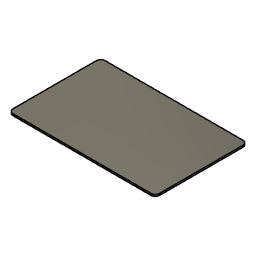
Part (Autodesk Fusion 360 archive; units mm, degrees)
design "Stainless_Steelx1mm_FacePlate"
Autodesk Fusion 360 part; units mm, degrees
sketch "Sketch1" plane through (0, 0, 0) normal (0, 1, 0) x (1, 0, 0)
  line L0 (40.5, -27) -> (-40.5, -27)
  line L1 (-43, -24.5) -> (-43, 24.5)
  line L2 (-40.5, 27) -> (40.5, 27)
  line L3 (43, 24.5) -> (43, -24.5)
  line L4 (43, -27) -> (-43, 27) construction
  line L5 (-43, -27) -> (43, 27) construction
  arc A0 (-40.5, 27) -> (-43, 24.5) centre (-40.5, 24.5) ccw
  arc A1 (43, 24.5) -> (40.5, 27) centre (40.5, 24.5) ccw
  arc A2 (40.5, -27) -> (43, -24.5) centre (40.5, -24.5) ccw
  arc A3 (-43, -24.5) -> (-40.5, -27) centre (-40.5, -24.5) ccw
  dimension "d1" = 86
  dimension "d2" = 54
  dimension "d5" = 2.5
  dimension "d6" = 2.5
  dimension "d7" = 2.5
  dimension "d8" = 2.5
  constraint horizontal L0
  constraint perpendicular L0 L1
  constraint parallel L0 L2
  constraint parallel L1 L3
  constraint coincident L4 origin
  constraint coincident L5 origin
  constraint coincident L4.end L1
  constraint coincident L4.end L2
  constraint tangent L1 A0
  constraint tangent L2 A0
  constraint coincident L5.end L2
  constraint coincident L5.end L3
  constraint tangent L2 A1
  constraint tangent L3 A1
  constraint coincident L4.start L3
  constraint coincident L4.start L0
  constraint tangent L3 A2
  constraint tangent L0 A2
  constraint coincident L5.start L0
  constraint coincident L5.start L1
  constraint tangent L0 A3
  constraint tangent L1 A3
  measures "d1" distance of L4.end L5.end
  measures "d2" distance of L5.start L4.end
  measures "d5" radius of A0
  measures "d6" radius of A1
  measures "d7" radius of A2
  measures "d8" radius of A3
extrude "Extrude1" add sketch "Sketch1" along normal blind 1

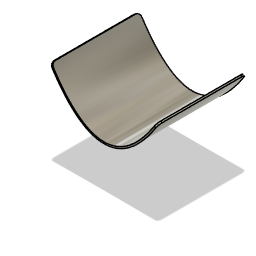
design "Stainless_Steelx1mm_CurvePlate"
Autodesk Fusion 360 part; units mm, degrees
sketch "Sketch1" plane through (0, 0, 0) normal (0, 0, 1) x (1, 0, 0)
  line L0 (0, 0) -> (32.17, 0) construction
  line L1 (0, 0) -> (0, -25.8728) construction
  line L2 (32.17, 0) -> (32.17, 25.8728) construction
  line L3 (-32.17, 25.8728) -> (-32.17, 0) construction
  line L4 (-32.17, 0) -> (0, 0) construction
  line L5 (-32.17, 25.8728) -> (0, -25.8728) construction
  line L6 (32.17, 25.8728) -> (0, -25.8728) construction
  spline S0 degree 2 poles (-32.17, 25.8728) (0, -25.8728) (32.17, 25.8728) knots 0 0 0 8.25666 8.25666 8.25666
  line L7 (0, 0) -> (0, 10)
  spline S1 degree 3 poles (-33.0193, 25.3448) (-25.8189, 13.763) (-18.5917, 5.9601) (-11.1994, 1.9953) (-5.2417, -1.2) (0.8588, -1.8451) (6.8666, 0.124) (14.6984, 2.6909) (22.3302, 9.5607) (29.9082, 20.5807) (30.9461, 22.0901) (31.9831, 23.6781) (33.0193, 25.3448) knots 0 0 0 0 2.75178 2.75178 2.75178 4.969537 4.969537 4.969537 7.860659 7.860659 7.860659 8.25666 8.25666 8.25666 8.25666
  line L8 (-32.17, 25.8728) -> (-33.0193, 25.3448)
  line L9 (33.0193, 25.3448) -> (32.17, 25.8728)
  dimension "d12" = 32.17
  dimension "d13" = 25.8728
  dimension "d14" = 25.8728
  dimension "d16" = 10
  dimension "d17" = 1
  constraint coincident L0.start L1.start
  constraint horizontal L0
  constraint perpendicular L0 L1
  constraint perpendicular L0 L2
  constraint symmetric L1 L2 L3
  constraint perpendicular L1 L4
  constraint equal L2 L3
  constraint coincident L1.end L5.end
  constraint perpendicular L0 L7
  constraint perpendicular L5 L8
  constraint perpendicular L6 L9
  measures "d12" distance of L0.start L0.end
  measures "d13" distance of L0.end L2.end
  measures "d14" distance of L0.start L1.end
  measures "d16" distance of L0.start L7.end
extrude "Extrude1" add sketch "Sketch1" along normal mid plane 54
fillet "Fillet1" radius 2.5 4 edges at (-32.5946, 25.6088, -27) (-32.5946, 25.6088, 27) (32.5946, 25.6088, 27) (32.5946, 25.6088, -27)
sketch "Sketch2" plane through (0, 0, 27) normal (0, 0, 1) x (1, 0, 0)
  line L0 (31.6793, 23.2341) -> (30.8299, 23.7622)
  spline S0 degree 2 poles (30.8299, 23.7622) (0, -23.7622) (-30.8299, 23.7622) knots -8.084689 -8.084689 -8.084689 -0.17197 -0.17197 -0.17197
  line L1 (-30.8299, 23.7622) -> (-31.6795, 23.234)
  spline S1 degree 3 poles (-31.6795, 23.234) (-24.922, 12.8101) (-18.1334, 5.7143) (-11.1994, 1.9953) (-5.2417, -1.2) (0.8588, -1.8451) (6.8666, 0.124) (14.6984, 2.6909) (22.3302, 9.5607) (29.9082, 20.5807) (30.4989, 21.4397) (31.0892, 22.3242) (31.6793, 23.2341) knots 0.170628 0.170628 0.170628 0.170628 2.75178 2.75178 2.75178 4.969537 4.969537 4.969537 7.860659 7.860659 7.860659 8.086023 8.086023 8.086023 8.086023
  point P0 (0, 10)
equation "xEnd = 32.17 mm"
equation "yEnd = 25.8728 mm"
equation "d12 = xEnd"
equation "d13 = yEnd"
equation "d14 = yEnd"
equation "d18 = 54 mm / 2"
